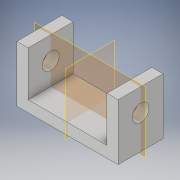
# Autodesk Inventor part: camPostHolderV02
Saved by Autodesk Inventor 2019.4 (Build 234330000, 330)
## iProperties
Created: 2019-04-27
Part Number: camPostHolderV02
Material: Generic
Document SubType Name: Modeling
Designer: steele
Density: 1 g/cm^3
Appearance: Default
Author: steele
Autodesk Inventor part; units mm, degrees
ref_plane "XZ Plane" through (0, 0, 0) normal (0, 1, 0) x (-1, 0, 0)
sketch "Sketch1" plane through (0, 0, 0) normal (0, 1, 0) x (-1, 0, 0)
  line L0 (28.575, 12.7) -> (-28.575, 12.7)
  line L1 (-28.575, 12.7) -> (-28.575, -12.7)
  line L2 (-28.575, -12.7) -> (28.575, -12.7)
  line L3 (28.575, -12.7) -> (28.575, 12.7)
  line L4 (28.575, 12.7) -> (-28.575, -12.7) construction
  line L5 (-28.575, 12.7) -> (28.575, -12.7) construction
  point P0 (0, 0)
  dimension "d0" = 57.15
  dimension "d1" = 25.4
  constraints: 12 end point, 2 midpoint, 2 parallel, 1 horizontal, 1 perpendicular
  measures "d0" distance of L0.start L0.end
  measures "d1" distance of L1.end L0.end
extrude "Extrusion1" add sketch "Sketch1" against normal blind 6.35
sketch "Sketch2" plane through (0, 0, 0) normal (0, 1, 0) x (1, 0, 0)
  line L0 (-28.575, -12.7) -> (-28.575, 12.7) projected
  line L1 (-28.575, -12.7) -> (-22.225, -12.7)
  line L2 (-22.225, -12.7) -> (-22.225, 12.7)
  line L3 (-22.225, 12.7) -> (-28.575, 12.7)
  line L4 (-28.575, 12.7) -> (-28.575, -12.7)
  point P0 (0, 0)
  dimension "d4" = 6.35
  constraints: 8 end point, 2 parallel, 1 horizontal, 1 perpendicular
  measures "d4" distance of L3.end L2.end
extrude "Extrusion2" add sketch "Sketch2" along normal blind 25.4
sketch "Sketch3" plane through (-28.575, -6.35, -12.7) normal (-1, 0, 0) x (0, 0, 1)
  circle A0 centre (12.7, 19.05) radius 4.7625
  line L0 (0, 31.75) -> (25.4, 31.75) projected
  circle A1 centre (12.7, -19.05) radius 4.0284
  point P0 (12.7, 6.35)
  dimension "d7" = 9.525
  dimension "d8" = 12.7
  dimension "d11" = 50.8
  constraints: 2 centre point
  measures "d7" diameter of A0
  measures "d8" distance from line of L0 A0.centre
  measures "d11" distance from line of A1.centre L0
extrude "Extrusion3" cut sketch "Sketch3" against normal through all contours A0
mirror "Mirror1" about plane through (0, 0, 0) normal (1, 0, 0) of "Extrusion2", "Extrusion3"
body "Solid1"
